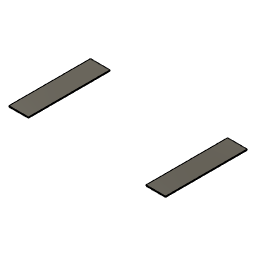
Stair Climber Motor Beds v5 (Autodesk Fusion 360 design; units mm, degrees)
Autodesk Fusion 360 part; units mm, degrees
sketch "Sketch1" plane through (0, 0, 0) normal (0, 0, 1) x (1, 0, 0)
  line L0 (240, 125) -> (-240, 125)
  line L1 (-240, 125) -> (-240, -125)
  line L2 (-240, -125) -> (240, -125)
  line L3 (240, -125) -> (240, 125)
  line L4 (240, 125) -> (-240, -125) construction
  line L5 (-240, 125) -> (240, -125) construction
  dimension "d1" = 480
  dimension "d2" = 250
  constraint horizontal L0
  constraint perpendicular L0 L1
  constraint parallel L0 L2
  constraint parallel L1 L3
  constraint coincident L4 origin
  constraint coincident L5 origin
  measures "d1" distance of L1.end L2.end
  measures "d2" distance of L0.end L1.end
extrude "Extrude1" add sketch "Sketch1" along normal blind 3 makes body 1
sketch "Sketch2" plane through (0, 0, 3) normal (0, 0, 1) x (-1, 0, 0)
  line L0 (-240, 125) -> (-240, -125)
  line L1 (-240, -125) -> (240, -125)
  line L2 (240, -125) -> (240, 125)
  line L3 (240, 125) -> (-240, 125)
  line L4 (0, 0) -> (210, 0) construction
  line L5 (0, 0) -> (-210, 0) construction
  line L6 (210, 0) -> (210, -125) construction
  line L7 (210, 0) -> (210, 125) construction
  line L8 (-210, 0) -> (-210, -125) construction
  line L9 (-210, 0) -> (-210, 125) construction
  dimension "d5" = 210
  dimension "d6" = 210
  constraint coincident L4.start L5.start
  constraint perpendicular L0 L4
  constraint perpendicular L0 L5
  constraint coincident L1 L6.end
  constraint perpendicular L1 L6
  constraint coincident L3 L7.end
  constraint perpendicular L3 L7
  constraint coincident L1 L8.end
  constraint perpendicular L1 L8
  constraint coincident L3 L9.end
  constraint perpendicular L3 L9
  measures "d5" distance of L4.start L4.end
  measures "d6" distance of L4.start L5.end
sketch "Sketch3" plane through (0, 0, 3) normal (0, 0, 1) x (-1, 0, 0)
  line L0 (210, 125) -> (180, 125) construction
  line L1 (180, 125) -> (180, -125) construction
  line L2 (180, -125) -> (210, -125) construction
  line L3 (210, -125) -> (210, 125) construction
  line L4 (-210, 125) -> (-180, 125) construction
  line L5 (-180, 125) -> (-180, -125) construction
  line L6 (-180, -125) -> (-210, -125) construction
  line L7 (-210, -125) -> (-210, 125) construction
  line L8 (180, -125) -> (-180, -125)
  line L9 (-180, -125) -> (-180, 125)
  line L10 (-180, 125) -> (180, 125)
  line L11 (180, 125) -> (180, -125)
  dimension "d7" = 30
  dimension "d8" = 250
  dimension "d9" = 30
  dimension "d10" = 250
  constraint horizontal L0
  constraint vertical L1
  constraint horizontal L2
  constraint vertical L3
  constraint horizontal L4
  constraint vertical L5
  constraint horizontal L6
  constraint vertical L7
  constraint horizontal L8
  constraint vertical L9
  constraint horizontal L10
  constraint vertical L11
  measures "d7" distance of L0.start L0.end
  measures "d8" distance of L0.start L2.end
  measures "d9" distance of L4.start L4.end
  measures "d10" distance of L4.start L6.end
extrude "Extrude2" cut sketch "Sketch3" against normal blind 20 bodies 1 makes body 2 at (200, 41.6667, 0)
sketch "Sketch4" plane through (0, 0, 3) normal (0, 0, 1) x (-1, 0, 0)
  line L0 (180, 125) -> (180, -125)
  line L1 (180, -125) -> (240, -125)
  line L2 (240, -125) -> (240, 125)
  line L3 (240, 125) -> (180, 125)
